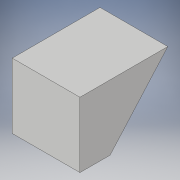
# Autodesk Inventor part: SouthEastWallBlockAngle
Saved by Autodesk Inventor 2018 (Build 220112000, 112)
## iProperties
Created: 2019-04-28
Part Number: SouthEastWallBlockAngle
Material: Generic
Document SubType Name: Modeling
Designer: snipe
Density: 1 g/cm^3
Appearance: Default
Author: snipe
Autodesk Inventor part; units mm, degrees
ref_plane "YZ Plane" through (0, 0, 0) normal (1, 0, 0) x (0, 1, 0)
ref_plane "XY Plane" through (0, 0, 0) normal (0, 0, 1) x (1, 0, 0)
sketch "Sketch1" plane through (0, 0, 0) normal (0, 1, 0) x (-1, 0, 0)
  line L0 (685.8, 304.8) -> (-685.8, 304.8)
  line L1 (-685.8, 304.8) -> (-685.8, -304.8)
  line L2 (-685.8, -304.8) -> (685.8, -304.8)
  line L3 (685.8, -304.8) -> (685.8, 304.8)
  line L4 (0, -426.72) -> (0, 426.72) projected
  line L5 (-960.12, 0) -> (960.12, 0) projected
  line L6 (960.12, 0) -> (-960.12, 0) projected
  line L7 (0, -426.72) -> (0, 426.72) projected
  point P0 (0, 0)
  dimension "d0" = 1371.6
  dimension "d1" = 609.6
  constraints: 8 end point, 2 parallel, 1 horizontal, 1 perpendicular, 2 other
  measures "d0" distance of L2.end L1.end
  measures "d1" distance of L1.end L0.end
ref_plane "Work Plane1" through (0, 1320.8, 0) normal (0, 1, 0) x (-1, 0, 0)
sketch "Sketch2" plane through (0, 1320.8, 0) normal (0, 1, 0) x (-1, 0, 0)
  line L0 (685.8, -304.8) -> (685.8, 304.8) projected
  line L1 (685.8, 304.8) -> (-685.8, 304.8) projected
  line L2 (685.8, 304.8) -> (-685.8, 304.8)
  line L3 (-685.8, 304.8) -> (-685.8, -1473.2)
  line L4 (-685.8, -1473.2) -> (685.8, -1473.2)
  line L5 (685.8, -1473.2) -> (685.8, 304.8)
  point P0 (0, 0)
  dimension "d3" = 1371.6
  dimension "d4" = 1778
  constraints: 8 end point, 2 parallel, 1 horizontal, 1 perpendicular
  measures "d3" distance of L4.end L3.end
  measures "d4" distance of L3.end L2.end
sketch "Sketch2 outline for Loft1" plane through (0, 1320.8, 0) normal (0, 1, 0) x (-1, 0, 0)
  line L0 (685.8, -1473.2) -> (685.8, 304.8)
  line L1 (-685.8, -1473.2) -> (685.8, -1473.2)
  line L2 (-685.8, 304.8) -> (-685.8, -1473.2)
  line L3 (685.8, 304.8) -> (-685.8, 304.8)
sketch "Sketch1 outline for Loft1" plane through (0, 0, 0) normal (0, 1, 0) x (-1, 0, 0)
  line L0 (685.8, -304.8) -> (685.8, 304.8)
  line L1 (-685.8, -304.8) -> (685.8, -304.8)
  line L2 (-685.8, 304.8) -> (-685.8, -304.8)
  line L3 (685.8, 304.8) -> (-685.8, 304.8)
loft "Loft1" add profiles "Sketch2 outline for Loft1", "Sketch1 outline for Loft1"
body "Solid1"
